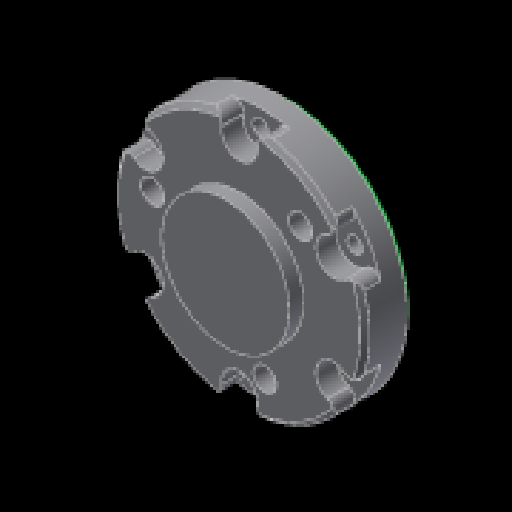
# Autodesk Inventor part: LegHub
Saved by Autodesk Inventor 2025.2 (Build 292293000, 293)
## iProperties
Created: 2025-10-14
Part Number: LegHub
Material: Generic
Document SubType Name: Modeling
Designer: valer
Density: 1 g/cm^3
Appearance: Default
Author: valer
Autodesk Inventor part; units mm, degrees
ref_plane "YZ Plane" through (0, 0, 0) normal (1, 0, 0) x (0, 1, 0)
ref_plane "XZ Plane" through (0, 0, 0) normal (0, 1, 0) x (-1, 0, 0)
ref_plane "XY Plane" through (0, 0, 0) normal (0, 0, 1) x (1, 0, 0)
sketch "Base" plane through (0, 0, 0) normal (0, 0, 1) x (1, 0, 0)
  circle A0 centre (14.2875, 0) radius 14.2875 projected
  circle A1 centre (34.9097, 11.9062) radius 1.9939 construction
  circle A2 centre (34.9097, -11.9063) radius 1.9939 construction
  circle A3 centre (14.2875, -23.8125) radius 1.9939 construction
  circle A4 centre (-6.3347, -11.9062) radius 1.9939 construction
  circle A5 centre (-6.3347, 11.9063) radius 1.9939 construction
  circle A6 centre (14.2875, 23.8125) radius 1.9939 construction
  circle A7 centre (14.2875, 0) radius 27.5127
  arc A8 (34.1709, -15.825) -> (37.934, -9.307) centre (34.9097, -11.9063) ccw construction
  circle A9 centre (-6.3347, 11.9063) radius 1.7272
  circle A10 centre (14.2875, 23.8125) radius 1.7272
  circle A11 centre (34.9097, 11.9062) radius 1.7272
  circle A12 centre (34.9097, -11.9063) radius 1.7272
  circle A13 centre (14.2875, -23.8125) radius 1.7272
  circle A14 centre (-6.3347, -11.9062) radius 1.7272
  point P0 (0, 0)
  dimension "d3" = 55.0254
  dimension "d10" = 3.4544
  constraints: 7 centre point, 7 coincident, 5 equal radius, 1 horizontal alignment
  measures "d3" diameter of A7
  measures "d10" diameter of A9
extrude "BaseFeature" add sketch "Base" along normal blind 10.3
sketch "SprocketMountHoles" plane through (14.2875, 0, 10.3) normal (0, 0, 1) x (1, 0, 0)
  circle A0 centre (5.5461, -18.6947) radius 3.175 construction
  circle A1 centre (13.417, 14.1504) radius 3.175 construction
  circle A2 centre (-18.9631, 4.5442) radius 3.175 construction
  circle A3 centre (-18.9631, 4.5442) radius 2.5527
  circle A4 centre (5.5461, -18.6947) radius 2.5527
  circle A5 centre (13.417, 14.1504) radius 2.5527
  point P0 (-14.2875, 0)
  dimension "d9" = 5.1054
  constraints: 3 centre point, 3 coincident, 2 equal radius
  measures "d9" diameter of A3
extrude "SprocketMountHolesFeature" cut sketch "SprocketMountHoles" against normal through all
chamfer "ChamfersFeature" distance 1 angle 45 2 edges at (-13.2252, 0, 0) (-13.2252, 0, 10.3)
sketch "Countersinks" plane through (14.2875, 0, 10.3) normal (0, 0, 1) x (1, 0, 0)
  circle A0 centre (-20.6222, 11.9063) radius 1.7272 construction
  circle A1 centre (0, 23.8125) radius 1.7272 construction
  circle A2 centre (20.6222, 11.9062) radius 1.7272 construction
  circle A3 centre (20.6222, -11.9063) radius 1.7272 construction
  circle A4 centre (0, -23.8125) radius 1.7272 construction
  circle A5 centre (-20.6222, -11.9062) radius 1.7272 construction
  circle A6 centre (-20.6222, 11.9063) radius 3.929
  circle A7 centre (0, 23.8125) radius 3.929
  circle A8 centre (20.6222, 11.9062) radius 3.929
  circle A9 centre (20.6222, -11.9063) radius 3.929
  circle A10 centre (0, -23.8125) radius 3.929
  circle A11 centre (-20.6222, -11.9062) radius 3.929
  point P0 (-14.2875, 0)
  dimension "d11" = 7.858
  constraints: 6 centre point, 6 coincident, 5 equal radius
  measures "d11" diameter of A6
extrude "CountersinksFeature" cut sketch "Countersinks" against normal blind 4.6656
fillet "CountersinkFilletsFeature" radius 2 12 edges at (-10.2173, -12.5086, 7.4672) (-8.7976, -14.9675, 7.4672) (-8.7976, 14.9675, 7.4672) (-10.2173, 12.5086, 7.4672) (12.8678, -27.476, 7.4672) (15.7072, -27.476, 7.4672) (37.3726, -14.9675, 7.4672) (38.7923, -12.5086, 7.4672) (38.7923, 12.5086, 7.4672) (37.3726, 14.9675, 7.4672) (15.7072, 27.476, 7.4672) (12.8678, 27.476, 7.4672)
ref_plane "ConnectPlane" through (-11.532, -25.8175, -6.5532) normal (0, 0, 1) x (0.8660254, 0.5, 0)
sketch "SprocketFlange" plane through (0, 0, 10.3) normal (0, 0, 1) x (1, 0, 0)
  arc A0 (18.6252, -26.1554) -> (34.7699, -16.8343) centre (14.2875, 0) ccw construction
  circle A1 centre (14.2875, 0) radius 14
  point P0 (0, 0)
  dimension "d20" = 28
  constraints: 1 centre point, 1 coincident
  measures "d20" diameter of A1
extrude "SprocketFlangeFeature" add sketch "SprocketFlange" along normal blind 3
sketch "WheelFlange" plane through (14.2875, 0, 0) normal (0, 0, -1) x (-1, 0, 0)
  circle A0 centre (0, 0) radius 14.2875 projected
  point P0 (14.2875, 0)
  constraints: 1 horizontal alignment
extrude "WheelFlangeFeature" add sketch "WheelFlange" against normal up to surface (10.3 mm away)
sketch "Sketch9" plane through (14.2875, 0, 0) normal (0, 0, -1) x (-1, 0, 0)
  circle A0 centre (0, 0) radius 26.5127 projected
  circle A1 centre (0, 0) radius 16.125
  point P0 (14.2875, 0)
  dimension "d30" = 32.25
  constraints: 1 centre point, 1 coincident
  measures "d30" diameter of A1
extrude "Extrusion9" cut sketch "Sketch9" against normal blind 3.25 contours A1
sketch "Sketch10" plane through (14.2875, 0, 3.25) normal (0, 0, -1) x (-1, 0, 0)
  circle A0 centre (0, 0) radius 16.125 projected
  circle A1 centre (0, 0) radius 14 projected
  circle A2 centre (0, 0) radius 4.165
  point P0 (14.2875, 0)
  dimension "d33" = 8.33
  constraints: 1 centre point, 1 coincident
  measures "d33" diameter of A2
extrude "Extrusion10" cut sketch "Sketch10" against normal through all contours A2
sketch "Sketch11" plane through (14.2875, 0, 3.25) normal (0, 0, -1) x (-1, 0, 0)
  circle A0 centre (8.4853, 8.4853) radius 2 construction
  circle A1 centre (-8.4853, 8.4853) radius 2 construction
  circle A2 centre (-8.4853, -8.4853) radius 2 construction
  circle A3 centre (8.4853, -8.4853) radius 2 construction
  circle A4 centre (8.4853, 8.4853) radius 1.7
  circle A5 centre (8.4853, -8.4853) radius 1.7
  circle A6 centre (-8.4853, 8.4853) radius 1.7
  circle A7 centre (-8.4853, -8.4853) radius 1.7
  point P0 (14.2875, 0)
  dimension "d36" = 4
  dimension "d37" = 3.4
  dimension "d38" = 3.4
  dimension "d39" = 3.4
  dimension "d40" = 3.4
  constraints: 8 centre point, 4 coincident, 8 other
  measures "d36" diameter of A0
  measures "d37" diameter of A4
  measures "d38" diameter of A5
  measures "d39" diameter of A6
  measures "d40" diameter of A7
extrude "Extrusion11" cut sketch "Sketch11" against normal blind 6
body "Solid1"
